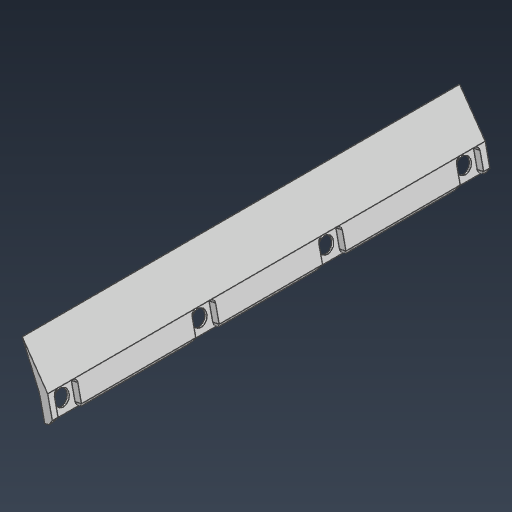
# Autodesk Inventor part: plog-uphold
Saved by Autodesk Inventor 2023 (Build 270158000, 158)
## iProperties
Created: 2025-07-08
Part Number: plog-uphold
Material: Generic
Document SubType Name: Modeling
Designer: szymo
Density: 1 g/cm^3
Appearance: Default
Author: szymo
Autodesk Inventor part; units mm, degrees
ref_plane "YZ Plane" through (0, 0, 0) normal (1, 0, 0) x (0, 1, 0)
ref_plane "XZ Plane" through (0, 0, 0) normal (0, 1, 0) x (-1, 0, 0)
ref_plane "XY Plane" through (0, 0, 0) normal (0, 0, 1) x (1, 0, 0)
sketch "Sketch1" plane through (0, 0, 0) normal (0, 0, 1) x (1, 0, 0)
  line L0 (-1.3868, -6.0009) -> (-1.1487, -7.998)
  line L1 (-1.1487, -7.998) -> (-0.7515, -7.9507)
  arc A0 (1.6124, -6.5682) -> (-0.7515, -7.9507) centre (1.9184, -9.8037) ccw
  line L2 (1.6124, -6.5682) -> (1.994, -6.4484)
  line L3 (1.994, -6.4484) -> (-2.7155, 8.55)
  line L4 (-2.7155, 8.55) -> (-3.1155, 8.5024)
  arc A1 (-0.8549, -10.1898) -> (2.172, -7.0153) centre (1.9184, -9.8037) ccw
  line L5 (1.994, -6.4484) -> (2.172, -7.0153)
  line L6 (1.994, -6.4484) -> (1.6124, -6.5682)
  arc A2 (1.6124, -6.5682) -> (-0.7515, -7.9507) centre (1.9184, -9.8037) ccw
  line L7 (-1.1487, -7.998) -> (-0.7515, -7.9507)
  line L8 (-1.0816, -8.5611) -> (-1.1487, -7.998)
  line L9 (-0.8549, -10.1898) -> (-1.0816, -8.5611)
  line L10 (-4.8217, 15.4245) -> (-4.165, 13.8337)
  line L11 (-4.8694, 15.4096) -> (-4.8217, 15.4245)
  line L12 (-4.8694, 15.4096) -> (0.523, -1.7637)
  line L13 (0.523, -1.7637) -> (0.7139, -1.7038)
  line L14 (-4.165, 13.8337) -> (0.7139, -1.7038)
  line L15 (0.7734, -6.2465) -> (1.9931, -5.9197)
  line L16 (-0.1066, -2.9624) -> (1.1131, -2.6356)
  line L17 (4.7729, -6.1987) -> (2.8198, -6.6293)
  line L18 (-2.2669, 7.7891) -> (1.6679, -1.4042)
  line L19 (1.6679, -1.4042) -> (2.8198, -6.6293)
  line L20 (-2.2669, 7.7891) -> (3.5145, -0.4906)
  line L21 (3.5145, -0.4906) -> (4.7729, -6.1987)
  line L22 (1.6679, -1.4042) -> (0.7139, -1.7038)
  line L23 (1.1131, -2.6356) -> (1.3264, -4.3221)
  line L24 (1.3264, -4.3221) -> (4.4133, -3.3528)
  line L25 (4.4133, -3.3528) -> (3.5145, -0.4906)
  line L26 (4.4133, -3.3528) -> (5.312, -6.2151)
  circle A3 centre (1.9184, -9.8037) radius 3.3
  circle A4 centre (1.9184, -9.8037) radius 1.9
  spline S0 degree 2 poles (-1.4487, -5.4815) (-1.4032, -5.7334) (-1.3868, -6.0009) knots 0 0 0 1 1 1 weights 1.291841 1.286703 1.276501
  line L27 (-3.1155, 8.5024) -> (-1.4487, -5.4815)
  point P0 (0, 0)
  dimension "d9" = 6.6
  dimension "d1" = 2
  dimension "d2" = 1
  dimension "d3" = 10
  dimension "d4" = 5
  dimension "d5" = 3.4
  dimension "d6" = 1.7
  dimension "d7" = 3
  dimension "d8" = 3
  constraints: 24 end point, 3 perpendicular, 1 coincident, 1 collinear, 1 parallel, 1 point on line, 12 other
  measures "d1" distance between parallel lines of L19 L21
  measures "d2" distance of L18.end L13.end
  measures "d3" distance of L18.start L18.end
  measures "d5" distance between parallel lines of L15 L16
  measures "d6" distance of L16.end L23.end
  measures "d7" distance of L20.end L24.end
  measures "d8" distance of L24.end L26.end
ref_plane "Work Plane1" through (-2.1629, -8.0975, -99) normal (0, 0, -1) x (0, 1, 0)
extrude "Extrusion1" add sketch "Sketch1" against normal up to surface (99 mm away) contours L19 L24 L21 L17 | L19 L18 L20 L21 L24
chamfer "Chamfer1" distance 1 angle 45 1 edges at (4.7729, -6.1987, -49.5) measured on face at (4.6653, -5.7104, -49.5)
fillet "Fillet2" radius 5 1 edges at (1.6679, -1.4042, -49.5)
ref_plane "Work Plane2" through (-2.4666, 7.7574, -28.025) normal (0.954071, 0.2995806, 0) x (-0.2995806, 0.954071, 0)
sketch "Sketch2" plane through (-2.4666, 7.7574, -28.025) normal (0.954071, 0.2995806, 0) x (-0.2995806, 0.954071, 0)
  circle A0 centre (-12.4265, -35.8125) radius 1.7 projected
  circle A1 centre (-12.4265, 24.025) radius 1.7 projected
  circle A2 centre (-12.4265, -7.1375) radius 1.7 projected
  circle A3 centre (-12.4265, -66.975) radius 1.7 projected
  line L0 (-14.8896, -42.65) -> (-14.8896, -70.975) projected
  line L1 (0.8308, -70.975) -> (-14.8896, -70.975) projected
  line L2 (0.8308, -70.975) -> (0.8308, 28.025) projected
  line L3 (-14.8896, 28.025) -> (0.8308, 28.025) projected
  line L4 (-14.8896, 28.025) -> (-14.8896, -0.3) projected
  line L5 (-14.8896, -0.3) -> (-15.4838, -0.3) projected
  line L6 (-15.4838, -0.3) -> (-15.4838, -13.975) projected
  line L7 (-15.4838, -42.65) -> (-14.8896, -42.65) projected
  line L8 (-15.4838, -13.975) -> (-14.5285, -13.975) projected
  line L9 (-14.5285, -28.975) -> (-15.4838, -28.975) projected
  line L10 (-15.4838, -28.975) -> (-15.4838, -42.65) projected
  line L11 (-14.5285, -13.975) -> (-14.5285, -28.975) projected
  point P0 (-8.14, 28.025)
extrude "Extrusion2" cut sketch "Sketch2" along normal up to surface contours A0 | A1 | A2 | A3 surface through (3.5145, -0.4906, 0) normal (0.9765506, 0.2152879, 0)
sketch "Sketch3" plane through (3.5145, -0.4906, 0) normal (0.9765506, 0.2152879, 0) x (0, 0, -1)
  line L0 (99, -4.8451) -> (99, 0) projected
  line L1 (0, 0) -> (99, 0) projected
  line L2 (0, -4.8451) -> (0, 0) projected
  line L3 (97.6, -5.7047) -> (92.3, -5.7047)
  line L4 (92.3, -5.7047) -> (92.3, 0)
  line L5 (92.3, 0) -> (97.6, 0)
  line L6 (97.6, 0) -> (97.6, -5.7047)
  line L7 (97.6, -5.7047) -> (92.3, 0) construction
  line L8 (92.3, -5.7047) -> (97.6, 0) construction
  line L9 (66.4375, -5.7047) -> (61.1375, -5.7047)
  line L10 (61.1375, -5.7047) -> (61.1375, 0)
  line L11 (61.1375, 0) -> (66.4375, 0)
  line L12 (66.4375, 0) -> (66.4375, -5.7047)
  line L13 (66.4375, -5.7047) -> (61.1375, 0) construction
  line L14 (61.1375, -5.7047) -> (66.4375, 0) construction
  line L15 (37.7625, -5.7047) -> (32.4625, -5.7047)
  line L16 (32.4625, -5.7047) -> (32.4625, 0)
  line L17 (32.4625, 0) -> (37.7625, 0)
  line L18 (37.7625, 0) -> (37.7625, -5.7047)
  line L19 (37.7625, -5.7047) -> (32.4625, 0) construction
  line L20 (32.4625, -5.7047) -> (37.7625, 0) construction
  line L21 (6.6, -5.7047) -> (1.3, -5.7047)
  line L22 (1.3, -5.7047) -> (1.3, 0)
  line L23 (1.3, 0) -> (6.6, 0)
  line L24 (6.6, 0) -> (6.6, -5.7047)
  line L25 (6.6, -5.7047) -> (1.3, 0) construction
  line L26 (1.3, -5.7047) -> (6.6, 0) construction
  line L27 (6.6, -5.7047) -> (1.3, -5.7047)
  line L28 (1.3, -5.7047) -> (1.3, -7.3492)
  line L29 (1.3, -7.3492) -> (6.6, -7.3492)
  line L30 (6.6, -7.3492) -> (6.6, -5.7047)
  line L31 (37.7625, -5.7047) -> (32.4625, -5.7047)
  line L32 (32.4625, -5.7047) -> (32.4625, -7.5222)
  line L33 (32.4625, -7.5222) -> (37.7625, -7.5222)
  line L34 (37.7625, -7.5222) -> (37.7625, -5.7047)
  line L35 (66.4375, -5.7047) -> (61.1375, -5.7047)
  line L36 (61.1375, -5.7047) -> (61.1375, -8.0969)
  line L37 (61.1375, -8.0969) -> (66.4375, -8.0969)
  line L38 (66.4375, -8.0969) -> (66.4375, -5.7047)
  line L39 (97.6, -5.7047) -> (92.3, -5.7047)
  line L40 (92.3, -5.7047) -> (92.3, -7.5222)
  line L41 (92.3, -7.5222) -> (97.6, -7.5222)
  line L42 (97.6, -7.5222) -> (97.6, -5.7047)
  line L43 (99, -4.8451) -> (0, -4.8451) projected
  point P0 (0, 1.2358)
  point P1 (63.7875, -2.8524)
  point P2 (3.95, -2.8524)
  point P3 (94.95, -2.8524)
  point P4 (35.1125, -2.8524)
  point P5 (6.6, 0)
  point P6 (37.7625, 0)
  point P7 (66.4375, 0)
  point P8 (97.6, 0)
  point P9 (1.3, -5.7047)
  dimension "d16" = 5.3
  dimension "d17" = 5.3
  dimension "d18" = 5.3
  dimension "d19" = 5.3
  constraints: 80 end point, 16 parallel, 8 horizontal, 8 midpoint, 8 perpendicular, 5 point on line
  measures "d16" distance of L4.end L5.end
  measures "d17" distance of L10.end L11.end
  measures "d18" distance of L16.end L17.end
  measures "d19" distance of L22.end L23.end
extrude "Extrusion3" cut sketch "Sketch3" against normal blind 1.5 contours L43 L4 L1 L6 | L6 L3 L4 L43 | L42 L41 L40 L3 | L43 L10 L1 L12 | L12 L9 L10 L43 | L38 L37 L36 L9 | L43 L16 L1 L18 | L18 L15 L16 L43 | L34 L33 L32 L15 | L43 L22 L1 L24 | L24 L21 L22 L43 | L30 L29 L28 L21
fillet "Fillet3" radius 1 16 edges at (2.7812, -0.6523, -97.6) (2.7812, -0.6523, -92.3) (2.7812, -0.6523, -66.4375) (2.7812, -0.6523, -61.1375) (2.7812, -0.6523, -37.7625) (2.7812, -0.6523, -32.4625) (2.7812, -0.6523, -1.3) (2.7812, -0.6523, -6.6) (3.5513, -6.468, -97.6) (3.5513, -6.468, -92.3) (3.5513, -6.468, -66.4375) (3.5513, -6.468, -61.1375) (3.5513, -6.468, -37.7625) (3.5513, -6.468, -32.4625) (3.5513, -6.468, -6.6) (3.5513, -6.468, -1.3)
equation "\"d6\" = 0.5 * d5"
equation "\"d17\" = d16"
equation "\"d18\" = d16"
equation "\"d19\" = d16"
body "Solid1"
